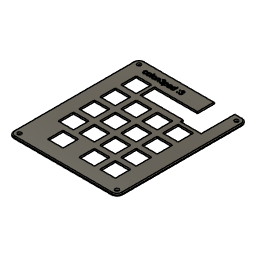
hackpad_case (Autodesk Fusion 360 archive; units mm, degrees)
design "Hackpad Plate"
Autodesk Fusion 360 part; units mm, degrees
sketch "Sketch1" plane through (0, 0, 0) normal (0, 0, 1) x (1, 0, 0)
  line L0 (3, -2.5) -> (16, -2.5)
  line L1 (3, -16.5) -> (16, -16.5)
  line L2 (2.5, -3) -> (2.5, -16)
  line L3 (16.5, -3) -> (16.5, -16)
  arc A0 (3, -2.5) -> (2.5, -3) centre (3, -3) ccw
  arc A1 (16.5, -3) -> (16, -2.5) centre (16, -3) ccw
  arc A2 (2.5, -16) -> (3, -16.5) centre (3, -16) ccw
  arc A3 (16, -16.5) -> (16.5, -16) centre (16, -16) ccw
  line L4 (3, -21.5) -> (16, -21.5)
  line L5 (3, -35.5) -> (16, -35.5)
  line L6 (2.5, -22) -> (2.5, -35)
  line L7 (16.5, -22) -> (16.5, -35)
  arc A4 (3, -21.5) -> (2.5, -22) centre (3, -22) ccw
  arc A5 (16.5, -22) -> (16, -21.5) centre (16, -22) ccw
  arc A6 (2.5, -35) -> (3, -35.5) centre (3, -35) ccw
  arc A7 (16, -35.5) -> (16.5, -35) centre (16, -35) ccw
  line L8 (22, -21.5) -> (35, -21.5)
  line L9 (22, -35.5) -> (35, -35.5)
  line L10 (21.5, -22) -> (21.5, -35)
  line L11 (35.5, -22) -> (35.5, -35)
  arc A8 (22, -21.5) -> (21.5, -22) centre (22, -22) ccw
  arc A9 (35.5, -22) -> (35, -21.5) centre (35, -22) ccw
  arc A10 (21.5, -35) -> (22, -35.5) centre (22, -35) ccw
  arc A11 (35, -35.5) -> (35.5, -35) centre (35, -35) ccw
  line L12 (41, -21.5) -> (54, -21.5)
  line L13 (41, -35.5) -> (54, -35.5)
  line L14 (40.5, -22) -> (40.5, -35)
  line L15 (54.5, -22) -> (54.5, -35)
  arc A12 (41, -21.5) -> (40.5, -22) centre (41, -22) ccw
  arc A13 (54.5, -22) -> (54, -21.5) centre (54, -22) ccw
  arc A14 (40.5, -35) -> (41, -35.5) centre (41, -35) ccw
  arc A15 (54, -35.5) -> (54.5, -35) centre (54, -35) ccw
  line L16 (60, -21.5) -> (73, -21.5)
  line L17 (60, -35.5) -> (73, -35.5)
  line L18 (59.5, -22) -> (59.5, -35)
  line L19 (73.5, -22) -> (73.5, -35)
  arc A16 (60, -21.5) -> (59.5, -22) centre (60, -22) ccw
  arc A17 (73.5, -22) -> (73, -21.5) centre (73, -22) ccw
  arc A18 (59.5, -35) -> (60, -35.5) centre (60, -35) ccw
  arc A19 (73, -35.5) -> (73.5, -35) centre (73, -35) ccw
  line L20 (3, -40.5) -> (16, -40.5)
  line L21 (3, -54.5) -> (16, -54.5)
  line L22 (2.5, -41) -> (2.5, -54)
  line L23 (16.5, -41) -> (16.5, -54)
  arc A20 (3, -40.5) -> (2.5, -41) centre (3, -41) ccw
  arc A21 (16.5, -41) -> (16, -40.5) centre (16, -41) ccw
  arc A22 (2.5, -54) -> (3, -54.5) centre (3, -54) ccw
  arc A23 (16, -54.5) -> (16.5, -54) centre (16, -54) ccw
  line L24 (22, -40.5) -> (35, -40.5)
  line L25 (22, -54.5) -> (35, -54.5)
  line L26 (21.5, -41) -> (21.5, -54)
  line L27 (35.5, -41) -> (35.5, -54)
  arc A24 (22, -40.5) -> (21.5, -41) centre (22, -41) ccw
  arc A25 (35.5, -41) -> (35, -40.5) centre (35, -41) ccw
  arc A26 (21.5, -54) -> (22, -54.5) centre (22, -54) ccw
  arc A27 (35, -54.5) -> (35.5, -54) centre (35, -54) ccw
  line L28 (41, -40.5) -> (54, -40.5)
  line L29 (41, -54.5) -> (54, -54.5)
  line L30 (40.5, -41) -> (40.5, -54)
  line L31 (54.5, -41) -> (54.5, -54)
  arc A28 (41, -40.5) -> (40.5, -41) centre (41, -41) ccw
  arc A29 (54.5, -41) -> (54, -40.5) centre (54, -41) ccw
  arc A30 (40.5, -54) -> (41, -54.5) centre (41, -54) ccw
  arc A31 (54, -54.5) -> (54.5, -54) centre (54, -54) ccw
  line L32 (60, -40.5) -> (73, -40.5)
  line L33 (60, -54.5) -> (73, -54.5)
  line L34 (59.5, -41) -> (59.5, -54)
  line L35 (73.5, -41) -> (73.5, -54)
  arc A32 (60, -40.5) -> (59.5, -41) centre (60, -41) ccw
  arc A33 (73.5, -41) -> (73, -40.5) centre (73, -41) ccw
  arc A34 (59.5, -54) -> (60, -54.5) centre (60, -54) ccw
  arc A35 (73, -54.5) -> (73.5, -54) centre (73, -54) ccw
  line L36 (3, -59.5) -> (16, -59.5)
  line L37 (3, -73.5) -> (16, -73.5)
  line L38 (2.5, -60) -> (2.5, -73)
  line L39 (16.5, -60) -> (16.5, -73)
  arc A36 (3, -59.5) -> (2.5, -60) centre (3, -60) ccw
  arc A37 (16.5, -60) -> (16, -59.5) centre (16, -60) ccw
  arc A38 (2.5, -73) -> (3, -73.5) centre (3, -73) ccw
  arc A39 (16, -73.5) -> (16.5, -73) centre (16, -73) ccw
  line L40 (22, -59.5) -> (35, -59.5)
  line L41 (22, -73.5) -> (35, -73.5)
  line L42 (21.5, -60) -> (21.5, -73)
  line L43 (35.5, -60) -> (35.5, -73)
  arc A40 (22, -59.5) -> (21.5, -60) centre (22, -60) ccw
  arc A41 (35.5, -60) -> (35, -59.5) centre (35, -60) ccw
  arc A42 (21.5, -73) -> (22, -73.5) centre (22, -73) ccw
  arc A43 (35, -73.5) -> (35.5, -73) centre (35, -73) ccw
  line L44 (41, -59.5) -> (54, -59.5)
  line L45 (41, -73.5) -> (54, -73.5)
  line L46 (40.5, -60) -> (40.5, -73)
  line L47 (54.5, -60) -> (54.5, -73)
  arc A44 (41, -59.5) -> (40.5, -60) centre (41, -60) ccw
  arc A45 (54.5, -60) -> (54, -59.5) centre (54, -60) ccw
  arc A46 (40.5, -73) -> (41, -73.5) centre (41, -73) ccw
  arc A47 (54, -73.5) -> (54.5, -73) centre (54, -73) ccw
  line L48 (60, -59.5) -> (73, -59.5)
  line L49 (60, -73.5) -> (73, -73.5)
  line L50 (59.5, -60) -> (59.5, -73)
  line L51 (73.5, -60) -> (73.5, -73)
  arc A48 (60, -59.5) -> (59.5, -60) centre (60, -60) ccw
  arc A49 (73.5, -60) -> (73, -59.5) centre (73, -60) ccw
  arc A50 (59.5, -73) -> (60, -73.5) centre (60, -73) ccw
  arc A51 (73, -73.5) -> (73.5, -73) centre (73, -73) ccw
  line L52 (12.5, -78.5) -> (25.5, -78.5)
  line L53 (12.5, -92.5) -> (25.5, -92.5)
  line L54 (12, -79) -> (12, -92)
  line L55 (26, -79) -> (26, -92)
  arc A52 (12.5, -78.5) -> (12, -79) centre (12.5, -79) ccw
  arc A53 (26, -79) -> (25.5, -78.5) centre (25.5, -79) ccw
  arc A54 (12, -92) -> (12.5, -92.5) centre (12.5, -92) ccw
  arc A55 (25.5, -92.5) -> (26, -92) centre (25.5, -92) ccw
  line L56 (4.062, -79.5) -> (10.062, -79.5)
  line L57 (4.062, -94.5) -> (10.062, -94.5)
  line L58 (3.562, -80) -> (3.562, -94)
  line L59 (10.562, -80) -> (10.562, -94)
  arc A56 (4.062, -79.5) -> (3.562, -80) centre (4.062, -80) ccw
  arc A57 (10.562, -80) -> (10.062, -79.5) centre (10.062, -80) ccw
  arc A58 (3.562, -94) -> (4.062, -94.5) centre (4.062, -94) ccw
  arc A59 (10.062, -94.5) -> (10.562, -94) centre (10.062, -94) ccw
  line L60 (27.938, -79.5) -> (33.938, -79.5)
  line L61 (27.938, -94.5) -> (33.938, -94.5)
  line L62 (27.438, -80) -> (27.438, -94)
  line L63 (34.438, -80) -> (34.438, -94)
  arc A60 (27.938, -79.5) -> (27.438, -80) centre (27.938, -80) ccw
  arc A61 (34.438, -80) -> (33.938, -79.5) centre (33.938, -80) ccw
  arc A62 (27.438, -94) -> (27.938, -94.5) centre (27.938, -94) ccw
  arc A63 (33.938, -94.5) -> (34.438, -94) centre (33.938, -94) ccw
  line L64 (41, -78.5) -> (54, -78.5)
  line L65 (41, -92.5) -> (54, -92.5)
  line L66 (40.5, -79) -> (40.5, -92)
  line L67 (54.5, -79) -> (54.5, -92)
  arc A64 (41, -78.5) -> (40.5, -79) centre (41, -79) ccw
  arc A65 (54.5, -79) -> (54, -78.5) centre (54, -79) ccw
  arc A66 (40.5, -92) -> (41, -92.5) centre (41, -92) ccw
  arc A67 (54, -92.5) -> (54.5, -92) centre (54, -92) ccw
  line L68 (60, -78.5) -> (73, -78.5)
  line L69 (60, -92.5) -> (73, -92.5)
  line L70 (59.5, -79) -> (59.5, -92)
  line L71 (73.5, -79) -> (73.5, -92)
  arc A68 (60, -78.5) -> (59.5, -79) centre (60, -79) ccw
  arc A69 (73.5, -79) -> (73, -78.5) centre (73, -79) ccw
  arc A70 (59.5, -92) -> (60, -92.5) centre (60, -92) ccw
  arc A71 (73, -92.5) -> (73.5, -92) centre (73, -92) ccw
  line L72 (-10.25, 12.75) -> (88.25, 12.75)
  line L73 (88.25, 12.75) -> (88.25, -105.75)
  line L74 (88.25, -105.75) -> (-10.25, -105.75)
  line L75 (-10.25, -105.75) -> (-10.25, 12.75)
  line L76 (3, -3) -> (16, -16) construction
  circle A72 centre (-5.25, 7.75) radius 1.7
  line L77 (39, 12.75) -> (39, -105.75) construction
  line L78 (-10.25, -46.5) -> (88.25, -46.5) construction
  circle A73 centre (83.25, 7.75) radius 1.7
  circle A74 centre (-5.25, -100.75) radius 1.7
  circle A75 centre (83.25, -100.75) radius 1.7
  line L79 (19.5, -2.9) -> (58.5, -2.9)
  line L80 (58.5, -2.9) -> (58.5, -15.9)
  line L81 (58.5, -15.9) -> (19.5, -15.9)
  line L82 (19.5, -15.9) -> (19.5, -2.9)
  line L83 (58.5, -18.5) -> (77.5, -18.5)
  line L84 (77.5, -18.5) -> (77.5, 12.75)
  line L85 (77.5, 12.75) -> (58.5, 12.75)
  line L86 (58.5, 12.75) -> (58.5, -18.5)
  point P0 (9.5, -9.5)
  dimension "d1" = 98.5
  dimension "d2" = 118.5
  dimension "d3" = 19.75
  dimension "d4" = 22.25
  dimension "d5" = 3.4
  dimension "d6" = 5
  dimension "d7" = 5
  dimension "d12" = 39
  dimension "d13" = 13
  dimension "d14" = 3
  dimension "d15" = 5.6
  dimension "d20" = 19
  dimension "d23" = 3
  constraint horizontal L72
  constraint vertical L73
  constraint horizontal L74
  constraint vertical L75
  constraint coincident A0.centre L76.start
  constraint coincident A3.centre L76.end
  constraint midpoint L76 P0
  constraint midpoint L72 L77.start
  constraint midpoint L74 L77.end
  constraint midpoint L75 L78.start
  constraint midpoint L73 L78.end
  constraint symmetric A72 L77 A73
  constraint symmetric A72 L78 A74
  constraint symmetric L78 A73 A75
  constraint horizontal L79
  constraint vertical L80
  constraint horizontal L81
  constraint vertical L82
  constraint horizontal L83
  constraint vertical L84
  constraint horizontal L85
  constraint vertical L86
  constraint coincident L79.end L86
  constraint coincident L72 L85.end
  measures "d1" distance of L72.start L72.end
  measures "d2" distance of L72.start L74.end
  measures "d3" distance of L75 P0
  measures "d4" distance of L72 P0
  measures "d5" diameter of A72
  measures "d6" distance of L72 A72.centre
  measures "d7" distance of L75 A72.centre
  measures "d12" distance of L79.start L79.end
  measures "d13" distance of L79.start L81.end
  measures "d14" distance of L3 L82
  measures "d15" distance of L8 L81
  measures "d20" distance of L83.start L83.end
  measures "d23" distance of L16 L83
extrude "Extrude1" add sketch "Sketch1" along normal blind 1.5 contours L56 L57 L58 L59 A56 A57 A58 A59 | L60 L61 L62 L63 A60 A61 A62 A63 | L72 L73 L74 L75 L79 L81 L82 L83 L84 L86
fillet "Fillet1" radius 5 4 edges at (88.25, -105.75, 0.75) (-10.25, -105.75, 0.75) (-10.25, 12.75, 0.75) (88.25, 12.75, 0.75)
sketch "Sketch2" plane through (0, 0, 1.5) normal (0, 0, 1) x (-1, 0, 0)
  arc A0 (-88.25, -7.75) -> (-83.25, -12.75) centre (-83.25, -7.75) ccw
  line L0 (-83.25, -12.75) -> (-77.5, -12.75)
  arc A1 (5.25, -12.75) -> (10.25, -7.75) centre (5.25, -7.75) ccw
  line L1 (10.25, -7.75) -> (10.25, 100.75)
  arc A2 (10.25, 100.75) -> (5.25, 105.75) centre (5.25, 100.75) ccw
  line L2 (5.25, 105.75) -> (-83.25, 105.75)
  arc A3 (-83.25, 105.75) -> (-88.25, 100.75) centre (-83.25, 100.75) ccw
  line L3 (-88.25, 100.75) -> (-88.25, -7.75)
  arc A4 (-41, 59.5) -> (-40.5, 60) centre (-41, 60) ccw
  line L4 (-41, 59.5) -> (-54, 59.5)
  arc A5 (-54.5, 60) -> (-54, 59.5) centre (-54, 60) ccw
  line L5 (-54.5, 60) -> (-54.5, 73)
  arc A6 (-54, 73.5) -> (-54.5, 73) centre (-54, 73) ccw
  line L6 (-54, 73.5) -> (-41, 73.5)
  arc A7 (-40.5, 73) -> (-41, 73.5) centre (-41, 73) ccw
  line L7 (-40.5, 73) -> (-40.5, 60)
  circle A8 centre (-83.25, -7.75) radius 1.7
  arc A9 (-12.5, 78.5) -> (-12, 79) centre (-12.5, 79) ccw
  line L8 (-12.5, 78.5) -> (-25.5, 78.5)
  arc A10 (-26, 79) -> (-25.5, 78.5) centre (-25.5, 79) ccw
  line L9 (-26, 79) -> (-26, 92)
  arc A11 (-25.5, 92.5) -> (-26, 92) centre (-25.5, 92) ccw
  line L10 (-25.5, 92.5) -> (-12.5, 92.5)
  arc A12 (-12, 92) -> (-12.5, 92.5) centre (-12.5, 92) ccw
  line L11 (-12, 92) -> (-12, 79)
  arc A13 (-41, 78.5) -> (-40.5, 79) centre (-41, 79) ccw
  line L12 (-41, 78.5) -> (-54, 78.5)
  arc A14 (-54.5, 79) -> (-54, 78.5) centre (-54, 79) ccw
  line L13 (-54.5, 79) -> (-54.5, 92)
  arc A15 (-54, 92.5) -> (-54.5, 92) centre (-54, 92) ccw
  line L14 (-54, 92.5) -> (-41, 92.5)
  arc A16 (-40.5, 92) -> (-41, 92.5) centre (-41, 92) ccw
  line L15 (-40.5, 92) -> (-40.5, 79)
  arc A17 (-3, 40.5) -> (-2.5, 41) centre (-3, 41) ccw
  line L16 (-3, 40.5) -> (-16, 40.5)
  arc A18 (-16.5, 41) -> (-16, 40.5) centre (-16, 41) ccw
  line L17 (-16.5, 41) -> (-16.5, 54)
  arc A19 (-16, 54.5) -> (-16.5, 54) centre (-16, 54) ccw
  line L18 (-16, 54.5) -> (-3, 54.5)
  arc A20 (-2.5, 54) -> (-3, 54.5) centre (-3, 54) ccw
  line L19 (-2.5, 54) -> (-2.5, 41)
  circle A21 centre (-83.25, 100.75) radius 1.7
  circle A22 centre (5.25, 100.75) radius 1.7
  arc A23 (-60, 40.5) -> (-59.5, 41) centre (-60, 41) ccw
  line L20 (-60, 40.5) -> (-73, 40.5)
  arc A24 (-73.5, 41) -> (-73, 40.5) centre (-73, 41) ccw
  line L21 (-73.5, 41) -> (-73.5, 54)
  arc A25 (-73, 54.5) -> (-73.5, 54) centre (-73, 54) ccw
  line L22 (-73, 54.5) -> (-60, 54.5)
  arc A26 (-59.5, 54) -> (-60, 54.5) centre (-60, 54) ccw
  line L23 (-59.5, 54) -> (-59.5, 41)
  arc A27 (-41, 21.5) -> (-40.5, 22) centre (-41, 22) ccw
  line L24 (-41, 21.5) -> (-54, 21.5)
  arc A28 (-54.5, 22) -> (-54, 21.5) centre (-54, 22) ccw
  line L25 (-54.5, 22) -> (-54.5, 35)
  arc A29 (-54, 35.5) -> (-54.5, 35) centre (-54, 35) ccw
  line L26 (-54, 35.5) -> (-41, 35.5)
  arc A30 (-40.5, 35) -> (-41, 35.5) centre (-41, 35) ccw
  line L27 (-40.5, 35) -> (-40.5, 22)
  line L28 (-58.5, 15.9) -> (-19.5, 15.9)
  line L29 (-19.5, 15.9) -> (-19.5, 2.9)
  line L30 (-19.5, 2.9) -> (-58.5, 2.9)
  arc A31 (-60, 59.5) -> (-59.5, 60) centre (-60, 60) ccw
  line L31 (-60, 59.5) -> (-73, 59.5)
  arc A32 (-73.5, 60) -> (-73, 59.5) centre (-73, 60) ccw
  line L32 (-73.5, 60) -> (-73.5, 73)
  arc A33 (-73, 73.5) -> (-73.5, 73) centre (-73, 73) ccw
  line L33 (-73, 73.5) -> (-60, 73.5)
  arc A34 (-59.5, 73) -> (-60, 73.5) centre (-60, 73) ccw
  line L34 (-59.5, 73) -> (-59.5, 60)
  arc A35 (-3, 2.5) -> (-2.5, 3) centre (-3, 3) ccw
  line L35 (-3, 2.5) -> (-16, 2.5)
  arc A36 (-16.5, 3) -> (-16, 2.5) centre (-16, 3) ccw
  line L36 (-16.5, 3) -> (-16.5, 16)
  arc A37 (-16, 16.5) -> (-16.5, 16) centre (-16, 16) ccw
  line L37 (-16, 16.5) -> (-3, 16.5)
  arc A38 (-2.5, 16) -> (-3, 16.5) centre (-3, 16) ccw
  line L38 (-2.5, 16) -> (-2.5, 3)
  arc A39 (-41, 40.5) -> (-40.5, 41) centre (-41, 41) ccw
  line L39 (-41, 40.5) -> (-54, 40.5)
  arc A40 (-54.5, 41) -> (-54, 40.5) centre (-54, 41) ccw
  line L40 (-54.5, 41) -> (-54.5, 54)
  arc A41 (-54, 54.5) -> (-54.5, 54) centre (-54, 54) ccw
  line L41 (-54, 54.5) -> (-41, 54.5)
  arc A42 (-40.5, 54) -> (-41, 54.5) centre (-41, 54) ccw
  line L42 (-40.5, 54) -> (-40.5, 41)
  arc A43 (-60, 78.5) -> (-59.5, 79) centre (-60, 79) ccw
  line L43 (-60, 78.5) -> (-73, 78.5)
  arc A44 (-73.5, 79) -> (-73, 78.5) centre (-73, 79) ccw
  line L44 (-73.5, 79) -> (-73.5, 92)
  arc A45 (-73, 92.5) -> (-73.5, 92) centre (-73, 92) ccw
  line L45 (-73, 92.5) -> (-60, 92.5)
  arc A46 (-59.5, 92) -> (-60, 92.5) centre (-60, 92) ccw
  line L46 (-59.5, 92) -> (-59.5, 79)
  arc A47 (-60, 21.5) -> (-59.5, 22) centre (-60, 22) ccw
  line L47 (-60, 21.5) -> (-73, 21.5)
  arc A48 (-73.5, 22) -> (-73, 21.5) centre (-73, 22) ccw
  line L48 (-73.5, 22) -> (-73.5, 35)
  arc A49 (-73, 35.5) -> (-73.5, 35) centre (-73, 35) ccw
  line L49 (-73, 35.5) -> (-60, 35.5)
  arc A50 (-59.5, 35) -> (-60, 35.5) centre (-60, 35) ccw
  line L50 (-59.5, 35) -> (-59.5, 22)
  arc A51 (-22, 59.5) -> (-21.5, 60) centre (-22, 60) ccw
  line L51 (-22, 59.5) -> (-35, 59.5)
  arc A52 (-35.5, 60) -> (-35, 59.5) centre (-35, 60) ccw
  line L52 (-35.5, 60) -> (-35.5, 73)
  arc A53 (-35, 73.5) -> (-35.5, 73) centre (-35, 73) ccw
  line L53 (-35, 73.5) -> (-22, 73.5)
  arc A54 (-21.5, 73) -> (-22, 73.5) centre (-22, 73) ccw
  line L54 (-21.5, 73) -> (-21.5, 60)
  arc A55 (-3, 21.5) -> (-2.5, 22) centre (-3, 22) ccw
  line L55 (-3, 21.5) -> (-16, 21.5)
  arc A56 (-16.5, 22) -> (-16, 21.5) centre (-16, 22) ccw
  line L56 (-16.5, 22) -> (-16.5, 35)
  arc A57 (-16, 35.5) -> (-16.5, 35) centre (-16, 35) ccw
  line L57 (-16, 35.5) -> (-3, 35.5)
  arc A58 (-2.5, 35) -> (-3, 35.5) centre (-3, 35) ccw
  line L58 (-2.5, 35) -> (-2.5, 22)
  arc A59 (-3, 59.5) -> (-2.5, 60) centre (-3, 60) ccw
  line L59 (-3, 59.5) -> (-16, 59.5)
  arc A60 (-16.5, 60) -> (-16, 59.5) centre (-16, 60) ccw
  line L60 (-16.5, 60) -> (-16.5, 73)
  arc A61 (-16, 73.5) -> (-16.5, 73) centre (-16, 73) ccw
  line L61 (-16, 73.5) -> (-3, 73.5)
  arc A62 (-2.5, 73) -> (-3, 73.5) centre (-3, 73) ccw
  line L62 (-2.5, 73) -> (-2.5, 60)
  arc A63 (-22, 40.5) -> (-21.5, 41) centre (-22, 41) ccw
  line L63 (-22, 40.5) -> (-35, 40.5)
  arc A64 (-35.5, 41) -> (-35, 40.5) centre (-35, 41) ccw
  line L64 (-35.5, 41) -> (-35.5, 54)
  arc A65 (-35, 54.5) -> (-35.5, 54) centre (-35, 54) ccw
  line L65 (-35, 54.5) -> (-22, 54.5)
  arc A66 (-21.5, 54) -> (-22, 54.5) centre (-22, 54) ccw
  line L66 (-21.5, 54) -> (-21.5, 41)
  arc A67 (-22, 21.5) -> (-21.5, 22) centre (-22, 22) ccw
  line L67 (-22, 21.5) -> (-35, 21.5)
  arc A68 (-35.5, 22) -> (-35, 21.5) centre (-35, 22) ccw
  line L68 (-35.5, 22) -> (-35.5, 35)
  arc A69 (-35, 35.5) -> (-35.5, 35) centre (-35, 35) ccw
  line L69 (-35, 35.5) -> (-22, 35.5)
  arc A70 (-21.5, 35) -> (-22, 35.5) centre (-22, 35) ccw
  line L70 (-21.5, 35) -> (-21.5, 22)
  circle A71 centre (5.25, -7.75) radius 1.7
  line L71 (-2.2743, -2.3244) -> (-54.284, -2.3883) construction
  line L72 (-54.284, -2.3883) -> (-54.2778, -7.3919) construction
  line L73 (-54.2778, -7.3919) -> (-2.2682, -7.328) construction
  line L74 (-2.2682, -7.328) -> (-2.2743, -2.3244) construction
  line L75 (-58.5, 18.5) -> (-58.5, 15.9)
  line L76 (-77.5, -12.75) -> (-77.5, 18.5)
  line L77 (-77.5, 18.5) -> (-58.5, 18.5)
  line L78 (-58.5, 2.9) -> (-58.5, -12.75)
  line L79 (-58.5, -12.75) -> (5.25, -12.75)
  dimension "d16" = 4.5
  text T0 "colon3pad :3" font "Arial" height 4.5 align left top in box 52.0097 x 5.0036 at (-2.2743, -2.3244) x (-0.999999, -0.001228) y (0.001228, -0.999999) spacing 1 kerned
extrude "Extrude2" cut sketch "Sketch2" against normal blind 0.2 text T0
fillet "Fillet2" radius 0.8 9 edges at (26.625, 12.75, 1.5) (-8.7855, 11.2855, 1.5) (-10.25, -46.5, 1.5) (-8.7855, -104.2855, 1.5) (39, -105.75, 1.5) (86.7855, -104.2855, 1.5) (88.25, -46.5, 1.5) (86.7855, 11.2855, 1.5) (80.375, 12.75, 1.5)
equation "d4 = 12.75 mm + 0.25 mm + 9.5 mm - 0.25 mm"
